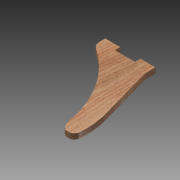
# Autodesk Inventor part: Pata
Saved by Autodesk Inventor 2015 (Build 190159000, 159)
## iProperties
Created: 2016-02-08
Part Number: Pata
Material: Wood (Birch)
Document SubType Name: Modeling
Designer: iberopuebla
Density: 0.55 g/cm^3
Appearance: Birch - Natural Polished
Author: iberopuebla
Autodesk Inventor part; units mm, degrees
ref_plane "YZ Plane" through (0, 0, 0) normal (1, 0, 0) x (0, 1, 0)
ref_plane "XZ Plane" through (0, 0, 0) normal (0, 1, 0) x (-1, 0, 0)
ref_plane "XY Plane" through (0, 0, 0) normal (0, 0, 1) x (1, 0, 0)
sketch "Sketch1" plane through (0, 0, 0) normal (0, 0, 1) x (1, 0, 0)
  arc A0 (176.5598, 33.6793) -> (12.6136, 287.2326) centre (-204.4335, -32.8889) ccw
  line L0 (167.9834, 291.8121) -> (218.9792, 109.3407)
  arc A1 (227.759, 27.1192) -> (218.9792, 109.3407) centre (-21.7947, 42.0509) ccw
  arc A2 (207.2823, -0.2492) -> (227.2466, 18.5563) centre (207.2823, 19.7508) ccw
  arc A3 (176.5598, 33.6793) -> (189.5473, 6.5592) centre (231.3648, 43.255) ccw
  arc A4 (189.5473, 6.5592) -> (204.58, -0.2492) centre (204.58, 19.7508) ccw
  line L1 (207.2823, -0.2492) -> (204.58, -0.2492)
  line L2 (227.759, 27.1192) -> (227.2466, 18.5563)
  arc A5 (248.2588, 303.6927) -> (197.3635, 355.4189) centre (196.5258, 303.6927) ccw
  line L3 (248.2588, 303.6927) -> (248.2588, 286.4547)
  arc A6 (222.3411, 252.6536) -> (248.2588, 286.4547) centre (213.2588, 286.4547) ccw
  line L4 (-281.6446, 363.1761) -> (197.3635, 355.4189)
  arc A7 (222.3411, 252.6536) -> (-337.0597, 3.3874) centre (731.561, -1642.4666) ccw
  line L5 (297.4263, 347.2322) -> (-473.2183, 347.2322) construction
  line L6 (-303.5209, 267.588) -> (-100.5419, 267.588)
  line L7 (-94.1908, 238.9989) -> (-285.5647, 149.5573)
  arc A8 (-94.1908, 238.9989) -> (-100.5419, 267.588) centre (-100.5419, 252.588) ccw
  arc A9 (-316.1527, 274.4986) -> (-303.5209, 267.588) centre (-303.5209, 282.588) ccw
  line L8 (-324.4601, 363.1761) -> (-281.6446, 363.1761)
  line L9 (-353.5533, 332.9002) -> (-316.1527, 274.4986)
  arc A10 (-324.4601, 363.1761) -> (-354.3192, 336.0808) centre (-324.4601, 333.1761) ccw
  arc A11 (-354.3192, 336.0808) -> (-353.5533, 332.9002) centre (-349.3427, 335.5967) ccw
  arc A12 (-358.3707, 23.1982) -> (-337.0597, 3.3874) centre (-345.2282, 15.9682) ccw
  line L10 (-292.3562, 143.1982) -> (-358.3707, 23.1982)
  arc A13 (-285.5647, 149.5573) -> (-292.3562, 143.1982) centre (-279.2137, 135.9682) ccw
  line L11 (-280.0505, 115.5231) -> (-264.2795, 106.8471)
  line L12 (-288.3795, 63.0385) -> (-264.2795, 106.8471)
  line L13 (-304.1505, 71.7145) -> (-288.3795, 63.0385)
  line L14 (-304.1505, 71.7145) -> (-280.0505, 115.5231)
  line L15 (-300.243, 286.193) -> (-282.243, 286.193)
  line L16 (-282.243, 336.193) -> (-300.243, 336.193)
  line L17 (-300.243, 336.193) -> (-300.243, 286.193)
  line L18 (199.757, 276.193) -> (181.757, 276.193)
  line L19 (181.757, 276.193) -> (181.757, 336.193)
  line L20 (181.757, 336.193) -> (199.757, 336.193)
  line L21 (199.757, 336.193) -> (199.757, 276.193)
  line L22 (-350.0834, 336.193) -> (288.2929, 336.193) construction
  line L23 (-282.243, 286.193) -> (-282.243, 336.193)
  line L24 (-194.243, 331.193) -> (-194.243, 313.193)
  line L25 (-94.243, 331.193) -> (-94.243, 313.193)
  line L26 (-194.243, 331.193) -> (-94.243, 331.193)
  line L27 (-94.243, 313.193) -> (-194.243, 313.193)
  line L28 (-282.243, 346.193) -> (-282.243, 276.193)
  line L29 (-282.243, 313.193) -> (-282.243, 331.193)
  line L30 (-282.243, 276.193) -> (-300.243, 276.193)
  line L31 (-300.243, 276.193) -> (-300.243, 346.193)
  line L32 (-300.243, 346.193) -> (-282.243, 346.193)
  line L33 (-6.243, 331.193) -> (-6.243, 313.193)
  line L34 (-6.243, 331.193) -> (93.757, 331.193)
  line L35 (93.757, 313.193) -> (-6.243, 313.193)
  line L36 (93.757, 331.193) -> (93.757, 313.193)
  line L37 (181.757, 331.193) -> (181.757, 313.193)
  line L38 (181.757, 346.193) -> (181.757, 266.193)
  line L39 (199.757, 346.193) -> (181.757, 346.193)
  line L40 (181.757, 266.193) -> (199.757, 266.193)
  line L41 (199.757, 266.193) -> (199.757, 346.193)
  line L42 (-0.5508, 312.0632) -> (-0.5508, 313.193)
  line L43 (166.8762, 299.8869) -> (166.8762, 313.193)
  line L44 (166.8762, 313.193) -> (-0.5508, 313.193)
  line L45 (166.8762, 313.193) -> (166.8762, 331.193)
  line L46 (166.8762, 331.193) -> (116.8762, 331.193)
  line L47 (116.8762, 331.193) -> (116.8762, 313.193)
  line L48 (-0.5508, 313.193) -> (-0.5508, 331.193)
  line L49 (-0.5508, 331.193) -> (49.4492, 331.193)
  line L50 (49.4492, 331.193) -> (49.4492, 313.193)
  arc A14 (-0.5508, 312.0632) -> (12.6136, 287.2326) centre (29.4492, 312.0632) ccw
  arc A15 (166.8762, 299.8869) -> (167.9834, 291.8121) centre (196.8762, 299.8869) ccw
  point P0 (0, 0)
  point P1 (-0.5508, 295.7736)
  point P2 (166.8762, 295.7736)
  point P3 (263.5097, 263.2389)
  point P4 (-311.7271, 267.588)
  point P5 (-289.9977, 147.4855)
  point P6 (-388.1512, -30.9362)
  point P7 (-291.243, 346.193)
  point P8 (372.0119, 346.193)
  dimension "d0" = 20
  dimension "d1" = 250
  dimension "d32" = 15
  dimension "d33" = 35
  dimension "d34" = 120
  dimension "d35" = 30
  dimension "d36" = 5
  dimension "d37" = 50
  dimension "d38" = 60
  dimension "d39" = 18
  dimension "d40" = 500
  dimension "d41" = 70
  dimension "d42" = 80
  dimension "d43" = 18
  dimension "d44" = 464
  dimension "d45" = 100
  dimension "d46" = 100
  dimension "d47" = 88
  dimension "d48" = 88
  dimension "d49" = 50
  dimension "d50" = 50
  dimension "d51" = 30
  dimension "d52" = 5.6922
  dimension "d53" = 67.427
  dimension "d54" = 30
  constraints: 102 end point, 35 point on circle, 26 tangent, 21 perpendicular, 16 centre point, 16 point on line, 14 parallel, 9 horizontal, 3 equal radius, 1 collinear, 1 vertical
  measures "d0" radius of A4
  measures "d1" radius of A1
  measures "d32" radius of A8
  measures "d33" radius of A6
  measures "d34" vertical distance of L10.start L10.end
  measures "d35" radius of A10
  measures "d36" radius of A11
  measures "d37" distance of L17.end L17.start
  measures "d38" distance of L20.end L18.start
  measures "d39" distance between parallel lines of L23 L17
  measures "d40" distance between parallel lines of L21 L17
  measures "d41" distance of L31.start L32.start
  measures "d42" distance of L38.end L38.start
  measures "d43" distance of L37.start L37.end
  measures "d44" distance of L29.end L37.start
  measures "d45" distance between parallel lines of L24 L25
  measures "d46" distance between parallel lines of L36 L33
  measures "d47" distance between parallel lines of L28 L24
  measures "d48" distance between parallel lines of L37 L36
  measures "d49" distance of L45.end L46.end
  measures "d50" distance of L48.end L49.end
  measures "d51" radius of A14
  measures "d52" distance between parallel lines of L33 L48
  measures "d53" distance between parallel lines of L47 L50
  measures "d54" radius of A15
extrude "Extrusion1" add sketch "Sketch1" along normal blind 18 contours A0 A7 L0 A1 L2 A2 L1 A4 A3 | A0 A14 L42 L35 L44 L43 A15 L0 A7
sketch "Sketch7" plane through (0, 0, 18) normal (0, 0, 1) x (1, 0, 0)
  line L0 (166.8762, 313.193) -> (166.8762, 331.193)
  line L1 (166.8762, 331.193) -> (116.8762, 331.193)
  line L2 (116.8762, 331.193) -> (116.8762, 313.193)
  line L3 (-0.5508, 313.193) -> (-0.5508, 331.193)
  line L4 (-0.5508, 331.193) -> (49.4492, 331.193)
  line L5 (49.4492, 331.193) -> (49.4492, 313.193)
  line L6 (166.8762, 313.193) -> (116.8762, 313.193)
  line L7 (49.4492, 313.193) -> (-0.5508, 313.193)
  point P0 (0, 0)
  dimension "d67" = 50
  dimension "d68" = 50
  dimension "d69" = 67.427
  constraints: 16 end point, 5 perpendicular, 1 parallel
  measures "d67" distance of L1.start L2.start
  measures "d68" distance of L3.end L4.end
  measures "d69" distance between parallel lines of L2 L5
extrude "Extrusion5" add sketch "Sketch7" against normal blind 18
sketch "Sketch8" plane through (0, 0, 18) normal (0, 0, 1) x (1, 0, 0)
  line L0 (195.4129, 0.9342) -> (223.5969, 0.9342)
  line L1 (223.5969, 0.9342) -> (223.5969, -9.3542)
  line L2 (223.5969, -9.3542) -> (195.4129, -9.3542)
  line L3 (195.4129, -9.3542) -> (195.4129, 0.9342)
  point P0 (0, 0)
  constraints: 8 end point, 2 parallel, 1 horizontal, 1 perpendicular
extrude "Extrusion6" cut sketch "Sketch8" against normal blind 18
body "Solid1"
